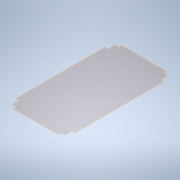
# Autodesk Inventor part: Robot bottom
Saved by Autodesk Inventor 2022 (Build 260153000, 153)
## iProperties
Created: 2023-01-13
Part Number: Robot bottom
Material: Polycarbonate, Smoke
Document SubType Name: Modeling
Designer: s135320
Mass: 3782.95 g
Surface Area: 10114.5 cm^2
Volume: 3152.46 cm^3
Density: 1.2 g/cm^3
Appearance: Polycarbonate - Smoked
Author: s135320
Autodesk Inventor part; units mm, degrees
ref_plane "YZ Plane" through (0, 0, 0) normal (1, 0, 0) x (0, 1, 0)
ref_plane "XZ Plane" through (0, 0, 0) normal (0, 1, 0) x (-1, 0, 0)
ref_plane "XY Plane" through (0, 0, 0) normal (0, 0, 1) x (1, 0, 0)
sketch "Sketch1" plane through (0, 0, 0) normal (0, 1, 0) x (-1, 0, 0)
  line L0 (0, 0) -> (-482.6, 0)
  line L1 (-482.6, 0) -> (-482.6, -889)
  line L2 (-482.6, -889) -> (0, -889)
  line L3 (0, -889) -> (0, 0)
  line L4 (0, -889) -> (-25.4, -889)
  line L5 (-25.4, -889) -> (-25.4, -806.45)
  line L6 (-25.4, -806.45) -> (0, -806.45)
  line L7 (0, -806.45) -> (0, -889)
  line L8 (-25.4, -889) -> (-57.15, -889)
  line L9 (-57.15, -889) -> (-57.15, -863.6)
  line L10 (-57.15, -863.6) -> (-25.4, -863.6)
  line L11 (-25.4, -863.6) -> (-25.4, -889)
  line L12 (-241.3, -889) -> (-241.3, -324.207) construction
  line L13 (0, -444.5) -> (-482.6, -444.5) construction
  line L14 (-457.2, -889) -> (-457.2, -806.45)
  line L15 (-457.2, -806.45) -> (-482.6, -806.45)
  line L16 (-425.45, -889) -> (-425.45, -863.6)
  line L17 (-425.45, -863.6) -> (-457.2, -863.6)
  line L18 (-25.4, 0) -> (-25.4, -82.55)
  line L19 (-25.4, -82.55) -> (0, -82.55)
  line L20 (-57.15, 0) -> (-57.15, -25.4)
  line L21 (-57.15, -25.4) -> (-25.4, -25.4)
  line L22 (-457.2, -82.55) -> (-482.6, -82.55)
  line L23 (-457.2, 0) -> (-457.2, -82.55)
  line L24 (-425.45, -25.4) -> (-457.2, -25.4)
  line L25 (-425.45, 0) -> (-425.45, -25.4)
  point P0 (-482.6, -82.55)
  point P1 (-482.6, -806.45)
  point P2 (0, -806.45)
  point P3 (0, -82.55)
  point P4 (-457.2, -25.4)
  dimension "d0" = 482.6
  dimension "d1" = 889
  dimension "d2" = 25.4
  dimension "d3" = 82.55
  dimension "d4" = 31.75
  dimension "d5" = 25.4
  constraints: 52 end point, 18 symmetric about line, 6 parallel, 3 horizontal, 3 midpoint, 3 perpendicular, 1 vertical
  measures "d0" distance of L2.end L1.end
  measures "d1" distance of L1.end L0.end
  measures "d2" distance of L5.end L6.end
  measures "d3" distance of L4.end L5.end
  measures "d4" distance of L9.end L10.end
  measures "d5" distance of L8.end L9.end
extrude "Extrusion1" add sketch "Sketch1" along normal blind 6.35 contours L3 L6 L5 L10 L9 L2 L16 L17 L14 L15 L1 L22 L23 L24 L25 L0 L20 L21 L18 L19
body "Solid1"
